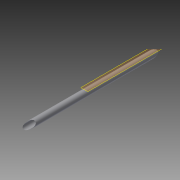
# Autodesk Inventor part: Launcher Crossbow
Saved by Autodesk Inventor 2014 SP1 (Build 180222100, 222)
## iProperties
Created: 2014-01-06
Part Number: Launcher Crossbow
Material: Generic
Document SubType Name: Modeling
Designer: Andrew Toennies
Density: 1 g/cm^3
Appearance: Default
Mass: 8.76691 g
Surface Area: 218.114 cm^2
Volume: 8.76691 cm^3
Author: Andrew Toennies
Autodesk Inventor part; units mm, degrees
ref_plane "YZ Plane" through (0, 0, 0) normal (1, 0, 0) x (0, 1, 0)
ref_plane "XY Plane" through (0, 0, 0) normal (0, 0, 1) x (1, 0, 0)
sketch "Sketch1" plane through (0, 0, 0) normal (0, 0, 1) x (1, 0, 0)
  circle A0 centre (0, 0) radius 6.35
  circle A1 centre (0, 0) radius 5.5372
  dimension "d0" = 12.7
  dimension "d1" = 11.0744
  constraints: 2 centre point, 2 coincident
  measures "d0" diameter of A0
  measures "d1" diameter of A1
extrude "Extrusion1" add sketch "Sketch1" along normal blind 304.8
ref_plane "Work Plane1" through (0, 6.35, 0) normal (0, 1, 0) x (-1, 0, 0)
sketch "Sketch2" plane through (0, 6.35, 0) normal (0, 1, 0) x (-1, 0, 0)
  circle A0 centre (0, 298.45) radius 1.5875
  line L0 (0, 298.45) -> (0, 0) construction
  dimension "d4" = 3.175
  dimension "d5" = 298.45
  constraints: 2 end point, 1 centre point, 1 vertical
  measures "d4" diameter of A0
  measures "d5" distance of L0.end L0.start
extrude "Extrusion2" cut sketch "Sketch2" against normal blind 25.4
ref_plane "Work Plane3" through (-1.1945, -6.2366, 0) normal (0.1881048, 0.982149, 0) x (-0.982149, 0.1881048, 0)
ref_plane "Work Plane2" through (-329.1366, 75.9683, 659.1579) normal (0.1881048, 0.982149, 0) x (-0.9818558, 0.1880487, -0.0244322)
sketch "Sketch3" plane through (-1.1945, -6.2366, 0) normal (0.1881048, 0.982149, 0) x (-0.982149, 0.1881048, 0)
  line L0 (0, 31.75) -> (0, 12.7) construction
  line L1 (-4.7625, 31.75) -> (-4.7625, 12.7)
  line L2 (4.7625, 12.7) -> (4.7625, 31.75)
  arc A0 (4.7625, 31.75) -> (-4.7625, 31.75) centre (0, 31.75) ccw
  arc A1 (-4.7625, 12.7) -> (4.7625, 12.7) centre (0, 12.7) ccw
  point P0 (0, 0)
  point P1 (0, 22.225)
  dimension "d10" = 9.525
  dimension "d11" = 19.05
  dimension "d12" = 12.7
  constraints: 8 end point, 4 point on circle, 4 tangent, 2 centre point, 1 midpoint, 1 parallel, 1 point on line, 1 vertical
  measures "d10" distance between parallel lines of L1 L2
  measures "d11" distance of L0.start L0.end
  measures "d12" distance of L0.end point (0, 0)
extrude "Extrusion3" cut sketch "Sketch3" along normal blind 25.4
body "Solid1"
